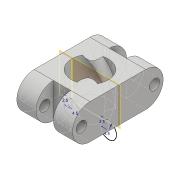
# Autodesk Inventor part: screw_nut
Saved by Autodesk Inventor 2018 (Build 220112000, 112)
## iProperties
Created: 2018-08-17
Part Number: screw_nut
Material: Generic
Document SubType Name: Modeling
Designer: Bardo91
Density: 1 g/cm^3
Appearance: Default
Author: Bardo91
Autodesk Inventor part; units mm, degrees
ref_plane "YZ Plane" through (0, 0, 0) normal (1, 0, 0) x (0, 1, 0)
ref_plane "XZ Plane" through (0, 0, 0) normal (0, 1, 0) x (-1, 0, 0)
ref_plane "XY Plane" through (0, 0, 0) normal (0, 0, 1) x (1, 0, 0)
sketch "Sketch1" plane through (0, 0, 0) normal (0, 0, 1) x (1, 0, 0)
  circle A0 centre (0, 0) radius 5.25
  line L0 (0, 0) -> (-8, 0)
  line L1 (-8, 0) -> (-8, 8)
  line L2 (-8, 8) -> (8, 8)
  line L3 (8, 8) -> (8, -8)
  line L4 (8, -8) -> (-8, -8)
  line L5 (-8, -8) -> (-8, 0)
  line L6 (0, -8) -> (-2.5, -8)
  line L7 (-2.5, -8) -> (-2.5, -13)
  line L8 (-2.5, -13) -> (-8, -13)
  line L9 (-8, -13) -> (-8, -8)
  line L10 (0, -8) -> (2.5, -8)
  line L11 (2.5, -8) -> (2.5, -13)
  line L12 (2.5, -13) -> (8, -13)
  line L13 (8, -13) -> (8, -8)
  line L14 (8, 0) -> (8, -2.5)
  line L15 (8, 0) -> (8, 2.5)
  line L16 (13, -2.5) -> (13, -8)
  line L17 (13, -8) -> (8, -8)
  line L18 (13, 2.5) -> (13, 8)
  line L19 (13, 8) -> (8, 8)
  line L20 (8, 2.5) -> (13, 2.5)
  line L21 (8, -2.5) -> (13, -2.5)
  line L22 (8, 8) -> (8, -8)
  line L23 (0, 8) -> (2.5, 8)
  line L24 (0, 8) -> (-2.5, 8)
  line L25 (2.5, 13) -> (8, 13)
  line L26 (8, 13) -> (8, 8)
  line L27 (-2.5, 13) -> (-8, 13)
  line L28 (-8, 13) -> (-8, 8)
  line L29 (-2.5, 8) -> (-2.5, 13)
  line L30 (2.5, 8) -> (2.5, 13)
  line L31 (-8, 8) -> (8, 8)
  line L32 (-8, 0) -> (-8, 2.5)
  line L33 (-8, 0) -> (-8, -2.5)
  line L34 (-13, 2.5) -> (-13, 8)
  line L35 (-13, 8) -> (-8, 8)
  line L36 (-13, -2.5) -> (-13, -8)
  line L37 (-13, -8) -> (-8, -8)
  line L38 (-8, -2.5) -> (-13, -2.5)
  line L39 (-8, 2.5) -> (-13, 2.5)
  line L40 (-8, -8) -> (-8, 8)
  dimension "d0" = 10.5
  dimension "d1" = 8
  dimension "d2" = 8
  dimension "d3" = 16
  dimension "d4" = 16
  dimension "d5" = 16
  dimension "d33" = 2.5
  dimension "d34" = 5
  dimension "d35" = 2.5
  dimension "d38" = 360
  constraints: 82 end point, 8 perpendicular, 8 point on line, 2 horizontal, 1 centre point, 1 coincident, 1 midpoint, 1 vertical, 73 other
  measures "d0" diameter of A0
  measures "d1" distance of L0.start L0.end
  measures "d2" distance of L0.end L1.end
  measures "d3" distance of L1.end L2.end
  measures "d4" distance of L2.end L3.end
  measures "d5" distance of L3.end L4.end
  measures "d33" distance of L6.start L6.end
  measures "d34" distance of L6.end L7.end
  measures "d35" distance of L6.start L10.end
extrude "Extrusion1" add sketch "Sketch1" along normal blind 10 contours L1 L2 L3 L4 L5 | L28 L27 L29 L2 | L4 L7 L8 L9 | L30 L25 L26 L2 | L4 L13 L12 L11
ref_plane "Work Plane1" through (-8, 0, 0) normal (0, -1, 0) x (1, 0, 0)
sketch "Sketch3" plane through (-8, 0, 0) normal (0, -1, 0) x (1, 0, 0)
  line L0 (13.3034, 0) -> (13.3034, -2.5)
  line L1 (2.75, 0) -> (2.75, 10) projected
  line L2 (2.75, 0) -> (2.75, -2.5)
  circle A0 centre (13.3034, -2.5) radius 2.25
  circle A1 centre (2.75, -2.5) radius 2.25
  point P0 (8, 0)
  dimension "d9" = 2.5
  dimension "d10" = 2.5
  dimension "d11" = 4.5
  dimension "d12" = 4.5
  constraints: 4 end point, 2 centre point, 2 coincident, 1 collinear, 1 point on line, 1 vertical
  measures "d9" distance of L0.start L0.end
  measures "d10" distance of L2.start L2.end
  measures "d11" diameter of A0
  measures "d12" diameter of A1
coil "Coil1" sketch "Sketch3" operation add axis through (0, 0, -10) along (0, 0, 1) pitch 35 turns 1 hand right contours A1
coil "Coil2" sketch "Sketch3" operation add axis through (0, 0, -10) along (0, 0, 1) pitch 35 turns 1 hand right contours A0
sketch "Sketch4" plane through (-8, -8, 0) normal (0, -1, 0) x (1, 0, 0)
  line L0 (10.5, 10) -> (5.5, 10) projected
  line L1 (0, 10) -> (16, 10)
  line L2 (16, 10) -> (16, 40)
  line L3 (16, 40) -> (0, 40)
  line L4 (0, 40) -> (0, 10)
  line L5 (10.5, 0) -> (5.5, 0) projected
  line L6 (0, 0) -> (16, 0)
  line L7 (16, 0) -> (16, -15)
  line L8 (16, -15) -> (0, -15)
  line L9 (0, -15) -> (0, 0)
  point P0 (8, 0)
  point P1 (16, 0)
  dimension "d29" = 30
  dimension "d30" = 15
  constraints: 16 end point, 4 parallel, 2 horizontal, 2 perpendicular, 1 point on line
  measures "d29" distance of L2.end L1.end
  measures "d30" distance of L6.end L7.end
extrude "Extrusion2" cut sketch "Sketch4" against normal through all
fillet "Fillet1" radius 5 8 edges at (5.25, -13, 10) (-5.25, -13, 10) (-5.25, 13, 10) (5.25, 13, 10) (-5.25, 13, 0) (5.25, 13, 0) (-5.25, -13, 0) (5.25, -13, 0)
sketch "Sketch6" plane through (8, -8, 0) normal (1, 0, 0) x (0, 0, -1)
  arc A0 (-10, 0) -> (0, 0) centre (-5, 0) ccw projected
  line L0 (-5, -5) -> (-5, -2.5)
  circle A1 centre (-5, -2.5) radius 1.5
  arc A2 (0, 16) -> (-10, 16) centre (-5, 16) ccw projected
  line L1 (-5, 21) -> (-5, 18.5)
  circle A3 centre (-5, 18.5) radius 1.5
  point P0 (0, 8)
  dimension "d41" = 2.5
  dimension "d42" = 3
  dimension "d43" = 2.5
  dimension "d44" = 3
  constraints: 4 end point, 2 centre point, 2 coincident, 2 point on circle, 2 vertical
  measures "d41" distance of L0.start L0.end
  measures "d42" diameter of A1
  measures "d43" distance of L1.start L1.end
  measures "d44" diameter of A3
extrude "Extrusion3" cut sketch "Sketch6" against normal through all
equation "\"d2\" = d1"
equation "\"d3\" = 2 * d1"
equation "\"d4\" = d3"
equation "\"d5\" = d3"
body "Solid1"
